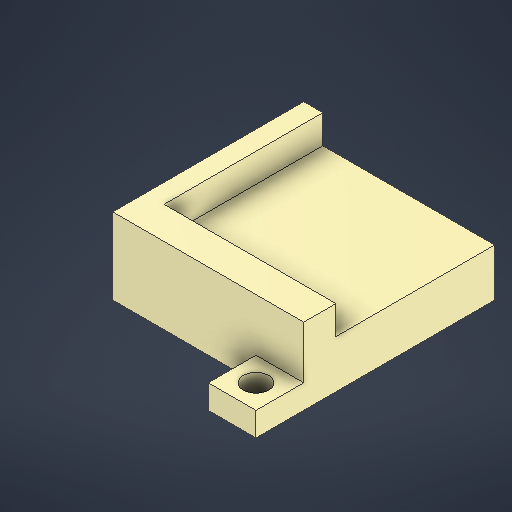
# Autodesk Inventor part: jetson_orin_nano_holder_corner_2
Saved by Autodesk Inventor 2026 (Build 300175050, 175E)
## iProperties
Created: 2025-06-11
Part Number: jetson_orin_nano_holder_corner_2
Material: Generic
Document SubType Name: Modeling
Designer: satom
Density: 1 g/cm^3
Appearance: Default
Author: satom
Autodesk Inventor part; units mm, degrees
ref_plane "YZ Plane" through (0, 0, 0) normal (1, 0, 0) x (0, 1, 0)
ref_plane "XZ Plane" through (0, 0, 0) normal (0, 1, 0) x (-1, 0, 0)
ref_plane "XY Plane" through (0, 0, 0) normal (0, 0, 1) x (1, 0, 0)
sketch "Sketch1" plane through (0, 0, 0) normal (0, 1, 0) x (-1, 0, 0)
  line L0 (0, 0) -> (96.52, 0)
  line L1 (96.52, 0) -> (96.52, -112.7)
  line L2 (96.52, -112.7) -> (0, -112.7)
  line L3 (0, -112.7) -> (0, 0)
  dimension "d0" = 96.52
  dimension "d1" = 112.7
  constraints: 8 end point, 2 parallel, 1 horizontal, 1 perpendicular
  measures "d0" distance of L0.start L0.end
  measures "d1" distance of L2.end L0.start
extrude "Extrusion1" add sketch "Sketch1" along normal blind 10.16
sketch "Sketch2" plane through (0, 10.16, 0) normal (0, 1, 0) x (1, 0, 0)
  line L0 (-96.52, 112.7) -> (-96.52, 0) construction
  line L1 (0, 0) -> (0, 112.7) construction
  line L2 (-96.52, 0) -> (0, 112.7) construction
  line L3 (0, 112.7) -> (-96.52, 112.7) construction
  line L4 (-96.52, 112.7) -> (0, 0) construction
  line L5 (-93.98, 4.28) -> (-2.54, 4.28)
  line L6 (-2.54, 4.28) -> (-2.54, 108.42)
  line L7 (-2.54, 108.42) -> (-93.98, 108.42)
  line L8 (-93.98, 108.42) -> (-93.98, 4.28)
  line L9 (-93.98, 4.28) -> (-2.54, 108.42) construction
  line L10 (-2.54, 4.28) -> (-93.98, 108.42) construction
  point P0 (-48.26, 56.35)
  dimension "d4" = 91.44
  dimension "d5" = 104.14
  constraints: 16 end point, 3 midpoint, 2 parallel, 1 horizontal, 1 perpendicular
  measures "d4" distance of L7.end L6.end
  measures "d5" distance of L5.end L6.end
extrude "Jetson Cavity" cut sketch "Sketch2" against normal blind 3.81
sketch "Sketch3" plane through (0, 0, 0) normal (0, -1, 0) x (1, 0, 0)
  line L0 (0, -19.05) -> (6.35, -19.05)
  line L1 (6.35, -19.05) -> (6.35, -25.4)
  line L2 (6.35, -25.4) -> (0, -25.4)
  circle A0 centre (3.175, -22.225) radius 1.7
  line L3 (6.35, -25.4) -> (0, -19.05) construction
  line L4 (6.35, -19.05) -> (0, -25.4) construction
  line L5 (0, 0) -> (0, -112.7) construction
  line L6 (0, -56.35) -> (-96.52, -56.35) construction
  line L7 (-96.52, -112.7) -> (-96.52, 0) construction
  line L8 (0, -112.7) -> (-96.52, -112.7) construction
  line L9 (-48.26, -112.7) -> (-48.26, 0) construction
  line L10 (-96.52, 0) -> (0, 0) construction
  line L11 (-96.52, 0) -> (-96.52, -112.7) construction
  line L12 (0, 0) -> (27.0549, 0) construction
  line L13 (0, -19.05) -> (0, -25.4)
  line L14 (-96.52, -19.05) -> (-102.87, -19.05)
  line L15 (-102.87, -19.05) -> (-102.87, -25.4)
  line L16 (-102.87, -25.4) -> (-96.52, -25.4)
  circle A1 centre (-99.695, -22.225) radius 1.7
  line L17 (-102.87, -25.4) -> (-96.52, -19.05) construction
  line L18 (-102.87, -19.05) -> (-96.52, -25.4) construction
  line L19 (-96.52, 0) -> (-96.52, -112.7) construction
  line L20 (-96.52, -19.05) -> (-96.52, -25.4)
  line L21 (0, -93.65) -> (6.35, -93.65)
  line L22 (6.35, -93.65) -> (6.35, -87.3)
  line L23 (6.35, -87.3) -> (0, -87.3)
  circle A2 centre (3.175, -90.475) radius 1.7
  line L24 (6.35, -87.3) -> (0, -93.65) construction
  line L25 (6.35, -93.65) -> (0, -87.3) construction
  line L26 (0, -112.7) -> (0, 0) construction
  line L27 (0, -93.65) -> (0, -87.3)
  line L28 (-96.52, -93.65) -> (-96.52, -87.3)
  circle A3 centre (-99.695, -90.475) radius 1.7
  line L29 (-102.87, -87.3) -> (-96.52, -93.65) construction
  line L30 (-102.87, -93.65) -> (-102.87, -87.3)
  line L31 (-102.87, -87.3) -> (-96.52, -87.3)
  line L32 (-102.87, -93.65) -> (-96.52, -87.3) construction
  line L33 (-96.52, -93.65) -> (-102.87, -93.65)
  line L34 (-77.47, 6.35) -> (-71.12, 6.35)
  line L35 (-71.12, 6.35) -> (-71.12, 0)
  line L36 (-71.12, 0) -> (-77.47, 0)
  line L37 (-77.47, 0) -> (-77.47, 6.35)
  line L38 (-77.47, 6.35) -> (-71.12, 0) construction
  line L39 (-71.12, 6.35) -> (-77.47, 0) construction
  circle A4 centre (-74.295, 3.175) radius 1.7
  line L40 (-96.52, 0) -> (-96.52, 26.4088) construction
  line L41 (-19.05, 6.35) -> (-25.4, 6.35)
  line L42 (-25.4, 6.35) -> (-25.4, 0)
  line L43 (-25.4, 0) -> (-19.05, 0)
  line L44 (-19.05, 0) -> (-19.05, 6.35)
  line L45 (-19.05, 6.35) -> (-25.4, 0) construction
  line L46 (-25.4, 6.35) -> (-19.05, 0) construction
  circle A5 centre (-22.225, 3.175) radius 1.7
  line L47 (-77.47, -119.05) -> (-71.12, -119.05)
  line L48 (-71.12, -119.05) -> (-71.12, -112.7)
  line L49 (-71.12, -112.7) -> (-77.47, -112.7)
  line L50 (-77.47, -112.7) -> (-77.47, -119.05)
  line L51 (-77.47, -119.05) -> (-71.12, -112.7) construction
  line L52 (-71.12, -119.05) -> (-77.47, -112.7) construction
  circle A6 centre (-74.295, -115.875) radius 1.7
  line L53 (-25.4, -112.7) -> (-19.05, -112.7)
  line L54 (-25.4, -119.05) -> (-25.4, -112.7)
  circle A7 centre (-22.225, -115.875) radius 1.7
  line L55 (-19.05, -112.7) -> (-19.05, -119.05)
  line L56 (-19.05, -119.05) -> (-25.4, -112.7) construction
  line L57 (-25.4, -119.05) -> (-19.05, -112.7) construction
  line L58 (-19.05, -119.05) -> (-25.4, -119.05)
  point P0 (-77.47, 3.175)
  point P1 (-19.05, 3.175)
  point P2 (-77.47, -115.875)
  point P3 (-19.05, -115.875)
  dimension "d10" = 3.4
  dimension "d28" = 6.35
  dimension "d29" = 6.35
  dimension "d30" = 19.05
  dimension "d31" = 6.35
  dimension "d32" = 6.35
  dimension "d33" = 3.4
  dimension "d34" = 19.05
  constraints: 110 end point, 38 symmetric about line, 8 centre point, 7 midpoint, 3 horizontal, 3 parallel, 2 perpendicular, 1 collinear, 1 vertical, 6 other
  measures "d10" diameter of A0
  measures "d28" distance of L0.end L1.end
  measures "d29" distance of L1.end L2.end
  measures "d30" distance between parallel lines of L12 L0
  measures "d31" distance of L35.end L36.end
  measures "d32" distance of L34.end L35.end
  measures "d33" diameter of A4
  measures "d34" distance from line of L40 point (-77.47, 3.175)
extrude "Screws" add sketch "Sketch3" against normal blind 3.175
sketch "Sketch5" plane through (0, 0, 0) normal (0, -1, 0) x (1, 0, 0)
  line L0 (-102.87, 6.35) -> (-71.12, 6.35)
  line L1 (-71.12, 6.35) -> (-71.12, -25.4)
  line L2 (-71.12, -25.4) -> (-102.87, -25.4)
  line L3 (-102.87, -25.4) -> (-102.87, 6.35)
  line L4 (-71.12, 6.35) -> (-77.47, 6.35) projected
  line L5 (-102.87, -19.05) -> (-102.87, -25.4) projected
  line L6 (-96.52, -19.05) -> (-96.52, 0) projected
  line L7 (-96.52, 0) -> (-77.47, 0) projected
  line L8 (-102.87, 6.35) -> (6.35, 6.35)
  line L9 (6.35, 6.35) -> (6.35, -119.05)
  line L10 (6.35, -119.05) -> (-102.87, -119.05)
  line L11 (-102.87, -119.05) -> (-102.87, 6.35)
  line L12 (6.35, -93.65) -> (6.35, -87.3) projected
  line L13 (-25.4, -119.05) -> (-19.05, -119.05) projected
  dimension "d35" = 25.4
  dimension "d36" = 25.4
  constraints: 16 end point, 4 collinear, 4 parallel, 2 horizontal, 2 perpendicular
  measures "d35" distance between parallel lines of L6 L1
  measures "d36" distance between parallel lines of L7 L2
extrude "Extrusion5" cut sketch "Sketch5" against normal through all contours L8 L9 L10 L11 L2 L1
equation "\"d10\" = m3_clearance"
equation "\"d33\" = m3_clearance"
equation "\"m3_heat_set_insert\" = 4"
equation "\"m3_clearance\" = 3.4"
equation "\"m3_heat_set_depth\" = 7"
equation "\"robot_diameter\" = 354"
equation "\"hardboard_thickness\" = 5"
body "Solid1"
